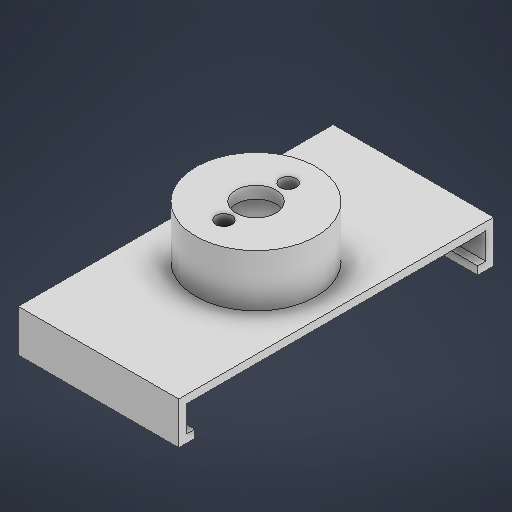
# Autodesk Inventor part: motor_prueba
Saved by Autodesk Inventor 2026 (Build 300175050, 175E)
## iProperties
Created: 2025-08-28
Part Number: motor_prueba
Material: Genérico
Document SubType Name: Modeling
Designer: rodri
Density: 1 g/cm^3
Appearance: Valor por defecto
Author: rodri
## iProperties of the stored document motor_prueba_3DPrint.ipt
Created: 2025-08-28
Part Number: motor_prueba_3DPrint
Material: Genérico
Document SubType Name: Modeling
Designer: rodri
Density: 1 g/cm^3
Appearance: Valor por defecto
Author: rodri
Autodesk Inventor part; units mm, degrees
ref_plane "YZ Plane" through (0, 0, 0) normal (1, 0, 0) x (0, 1, 0)
ref_plane "XZ Plane" through (0, 0, 0) normal (0, 1, 0) x (-1, 0, 0)
ref_plane "XY Plane" through (0, 0, 0) normal (0, 0, 1) x (1, 0, 0)
sketch "Boceto1" plane through (0, 0, 0) normal (0, 1, 0) x (-1, 0, 0)
  circle A0 centre (0, 0) radius 15
  circle A1 centre (0, 0) radius 5
  circle A2 centre (0, 8) radius 2
  circle A3 centre (0, -8) radius 2
  dimension "d0" = 30
  dimension "d1" = 10
  dimension "d2" = 4
  dimension "d3" = 8
  dimension "d4" = 4
  dimension "d5" = 8
  constraints: 4 centre point, 2 coincident
  measures "d0" diameter of A0
  measures "d1" diameter of A1
  measures "d2" diameter of A2
  measures "d3" distance of A2.centre point (0, 0)
  measures "d4" diameter of A3
  measures "d5" distance of A3.centre point (0, 0)
extrude "Extrusión1" add sketch "Boceto1" against normal blind 3
sketch "Boceto2" plane through (0, -3, 0) normal (0, -1, 0) x (1, 0, 0)
  circle A0 centre (0, 0) radius 11
  circle A1 centre (0, 0) radius 15
  dimension "d8" = 22
  constraints: 2 centre point, 2 coincident
  measures "d8" diameter of A0
extrude "Extrusión2" add sketch "Boceto2" along normal blind 10
sketch "Boceto5" plane through (0, 0, 0) normal (1, 0, 0) x (0, 1, 0)
  line L0 (-15, 0) -> (-15, 37.25)
  line L1 (-32.5779, 0) -> (6.5779, 0) construction
  line L2 (-13, 39.25) -> (-13, 0)
  line L3 (-13, 39.25) -> (-23.5, 39.25)
  line L4 (-23.5, 39.25) -> (-23.5, 35.25)
  line L5 (-23.5, 35.25) -> (-21.5, 35.25)
  line L6 (-21.5, 35.25) -> (-21.5, 37.25)
  line L7 (-21.5, 37.25) -> (-15, 37.25)
  line L8 (-15, 0) -> (-15, -37.25)
  line L9 (-13, -39.25) -> (-13, 0)
  line L10 (-13, -39.25) -> (-23.5, -39.25)
  line L11 (-23.5, -39.25) -> (-23.5, -35.25)
  line L12 (-23.5, -35.25) -> (-21.5, -35.25)
  line L13 (-21.5, -35.25) -> (-21.5, -37.25)
  line L14 (-21.5, -37.25) -> (-15, -37.25)
  point P0 (0, 0)
  dimension "d27" = 10.5
  dimension "d28" = 4
  dimension "d29" = 2
  dimension "d30" = 2
  constraints: 30 end point, 6 symmetric about line, 3 perpendicular, 2 horizontal, 1 midpoint, 1 parallel, 1 point on line
  measures "d27" distance of L2.start L3.end
  measures "d28" distance of L3.end L4.end
  measures "d29" distance of L4.end L5.end
  measures "d30" distance of L5.end L6.end
extrude "Extrusión5" add sketch "Boceto5" along normal mid plane 40
sketch "Boceto6" plane through (0, -13, 0) normal (0, 1, 0) x (1, 0, 0)
  circle A0 centre (0, 0) radius 11 projected
  point P0 (0, 0)
extrude "Extrusión6" cut sketch "Boceto6" against normal through all
